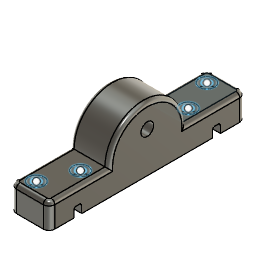
ersatzteilTischtennisplatte (Autodesk Fusion 360 design; units mm, degrees)
part number: 2025-12-14-13-54-51-674
Autodesk Fusion 360 part; units mm, degrees
sketch "Skizze1" plane through (0, 0, 0) normal (1, 0, 0) x (0, 1, 0)
  line L0 (0, 0) -> (51, 0)
  line L1 (0, 0) -> (-51, 0)
  line L2 (-51, 0) -> (-51, 13)
  line L3 (51, 0) -> (51, 13)
  line L4 (51, 13) -> (20, 13)
  line L5 (-51, 13) -> (-20, 13)
  arc A0 (20, 13) -> (-20, 13) centre (0, 13) ccw
  line L6 (-51, 0) -> (-38, 0)
  line L7 (51, 0) -> (38, 0)
  dimension "d6" = 13
  dimension "d10" = 51
  dimension "d11" = 40
  dimension "d12" = 13
  dimension "d13" = 13
  constraint coincident L0.start L1.start
  constraint horizontal L0
  constraint parallel L0 L1
  constraint perpendicular L1 L2
  constraint perpendicular L0 L3
  constraint perpendicular L3 L4
  constraint perpendicular L2 L5
  constraint perpendicular L2 L6
  constraint perpendicular L3 L7
  measures "d6" distance of L1.end L2.end
  measures "d10" distance of L0.start L0.end
  measures "d11" diameter of A0
  measures "d12" distance of L1.end L6.end
  measures "d13" distance of L0.end L7.end
extrude "Extrusion1" add sketch "Skizze1" along normal blind 20
fillet "Abrundung1" radius 2 8 edges at (10, -51, 13) (20, -35.5, 13) (0, -35.5, 13) (20, 0, 33) (0, 0, 33) (0, 35.5, 13) (20, 35.5, 13) (10, 51, 13)
fillet "Abrundung2" radius 3 8 edges at (0, 51, 5.5) (0.5858, 50.4142, 12.4142) (20, 51, 5.5) (19.4142, 50.4142, 12.4142) (19.4142, -50.4142, 12.4142) (20, -51, 5.5) (0, -51, 5.5) (0.5858, -50.4142, 12.4142)
sketch "Skizze2" plane through (20, 0, 0) normal (1, 0, 0) x (0, 1, 0)
  line L0 (-48, 11) -> (-48, 0)
  line L1 (-48, 0) -> (48, 0)
  line L2 (48, 0) -> (48, 11)
  line L3 (48, 11) -> (17.8885, 11)
  arc A0 (17.8885, 11) -> (-17.8885, 11) centre (0, 13) ccw
  line L4 (-17.8885, 11) -> (-48, 11)
  circle A1 centre (0, 21) radius 3.3
  dimension "d22" = 21
  dimension "d23" = 6.6
  measures "d22" distance of origin A1.centre
  measures "d23" diameter of A1
extrude "Extrusion2" cut sketch "Skizze2" against normal blind 100 contours A1
sketch "Skizze3" plane through (0, 0, 0) normal (-1, 0, 0) x (0, -1, 0)
  circle A0 centre (0, 21) radius 3.3
  line L0 (48, 0) -> (48, 11)
  line L1 (48, 11) -> (17.8885, 11)
  arc A1 (17.8885, 11) -> (-17.8885, 11) centre (0, 13) ccw
  line L2 (-17.8885, 11) -> (-48, 11)
  line L3 (-48, 11) -> (-48, 0)
  line L4 (-48, 0) -> (48, 0)
  line L5 (-6, 17.5359) -> (0, 14.0718)
  line L6 (0, 14.0718) -> (6, 17.5359)
  line L7 (6, 17.5359) -> (6, 24.4641)
  line L8 (6, 24.4641) -> (0, 27.9282)
  line L9 (0, 27.9282) -> (-6, 24.4641)
  line L10 (-6, 24.4641) -> (-6, 17.5359)
  point P0 (0, 21)
  dimension "d26" = 6
  constraint coincident P0 A0.centre
  measures "d26" distance of P0 L10
extrude "Extrusion3" cut sketch "Skizze3" against normal blind 6 contours L5 L6 L7 L8 L9 L10
sketch "Skizze4" plane through (0, 0, 0) normal (-1, 0, 0) x (0, -1, 0)
  line L0 (0, 14.0718) -> (-6, 17.5359)
  line L1 (-6, 17.5359) -> (-6, 24.4641)
  line L2 (-6, 24.4641) -> (0, 27.9282)
  line L3 (0, 27.9282) -> (6, 24.4641)
  line L4 (6, 24.4641) -> (6, 17.5359)
  line L5 (6, 17.5359) -> (0, 14.0718)
  line L6 (48, 0) -> (48, 11)
  line L7 (48, 11) -> (17.8885, 11)
  arc A0 (17.8885, 11) -> (-17.8885, 11) centre (0, 13) ccw
  line L8 (-17.8885, 11) -> (-48, 11)
  line L9 (-48, 11) -> (-48, 0)
  line L10 (-48, 0) -> (48, 0)
  line L11 (51, 0) -> (38, 0)
  line L12 (-51, 0) -> (-38, 0)
  line L13 (-38, 0) -> (-38, 4.8)
  line L14 (-38, 4.8) -> (-34, 4.8)
  line L15 (-34, 4.8) -> (-34, 0)
  dimension "d29" = 13
  dimension "d30" = 13
  dimension "d31" = 4.8
  dimension "d32" = 4
  constraint perpendicular L6 L11
  constraint perpendicular L9 L12
  constraint perpendicular L10 L13
  constraint perpendicular L13 L14
  constraint coincident L10 L15.end
  constraint perpendicular L10 L15
  measures "d29" distance of L11.start L11.end
  measures "d30" distance of L12.start L12.end
  measures "d31" distance of L12.end L13.end
  measures "d32" distance of L13.end L14.end
extrude "Extrusion4" cut sketch "Skizze4" against normal blind 100 contours L10 L13 L14 L15
fillet "Abrundung3" radius 1 2 edges at (10, 34, 4.8) (10, 38, 4.8)
sketch "Skizze5" plane through (0, 0, 0) normal (-1, 0, 0) x (0, -1, 0)
  line L0 (-34, 3.8) -> (-34, 0)
  line L1 (-34, 0) -> (48, 0)
  line L2 (48, 0) -> (48, 11)
  line L3 (48, 11) -> (17.8885, 11)
  arc A0 (17.8885, 11) -> (-17.8885, 11) centre (0, 13) ccw
  line L4 (-17.8885, 11) -> (-48, 11)
  line L5 (-48, 11) -> (-48, 0)
  line L6 (-48, 0) -> (-38, 0)
  line L7 (-38, 0) -> (-38, 3.8)
  arc A1 (-37, 4.8) -> (-38, 3.8) centre (-37, 3.8) ccw
  line L8 (-37, 4.8) -> (-35, 4.8)
  arc A2 (-34, 3.8) -> (-35, 4.8) centre (-35, 3.8) ccw
  line L9 (0, 14.0718) -> (-6, 17.5359)
  line L10 (-6, 17.5359) -> (-6, 24.4641)
  line L11 (-6, 24.4641) -> (0, 27.9282)
  line L12 (0, 27.9282) -> (6, 24.4641)
  line L13 (6, 24.4641) -> (6, 17.5359)
  line L14 (6, 17.5359) -> (0, 14.0718)
  line L15 (51, 0) -> (38, 0)
  line L16 (38, 0) -> (38, 4.8)
  line L17 (38, 4.8) -> (34, 4.8)
  line L18 (34, 4.8) -> (34, 0)
  dimension "d37" = 13
  dimension "d38" = 4.8
  dimension "d39" = 4
  constraint perpendicular L2 L15
  constraint perpendicular L1 L16
  constraint perpendicular L16 L17
  constraint coincident L1 L18.end
  constraint perpendicular L1 L18
  measures "d37" distance of L15.start L15.end
  measures "d38" distance of L15.end L16.end
  measures "d39" distance of L16.end L17.end
extrude "Extrusion5" cut sketch "Skizze5" against normal blind 100 contours L1 L16 L17 L18
fillet "Abrundung4" radius 1 2 edges at (10, -34, 4.8) (10, -38, 4.8)
sketch "Skizze6" plane through (0, 0, 13) normal (0, 0, 1) x (-1, 0, 0)
  arc A0 (-18, -48) -> (-17, -49) centre (-17, -48) ccw
  line L0 (-17, -49) -> (-3, -49)
  arc A1 (-3, -49) -> (-2, -48) centre (-3, -48) ccw
  line L1 (-2, -48) -> (-2, -20)
  line L2 (-2, -20) -> (-18, -20)
  line L3 (-18, -20) -> (-18, -48)
  circle A2 centre (-6.7, 44.3) radius 2.15
  circle A3 centre (-13.3, 28) radius 2.15
  circle A4 centre (-13.3, -28) radius 2.15
  circle A5 centre (-6.7, -44.3) radius 2.15
  circle A6 centre (-13.3, 28) radius 4
  circle A7 centre (-6.7, 44.3) radius 4
  circle A8 centre (-13.3, -28) radius 4
  circle A9 centre (-6.7, -44.3) radius 4
  dimension "d55" = 4.3
  dimension "d58" = 4.3
  dimension "d61" = 8
  dimension "d62" = 8
  dimension "d63" = 8
  dimension "d64" = 8
  dimension "d67" = 4.3
  dimension "d68" = 4.3
  constraint concentric A3 A6
  constraint concentric A2 A7
  constraint concentric A4 A8
  constraint concentric A5 A9
  measures "d55" diameter of A2
  measures "d58" diameter of A3
  measures "d61" diameter of A6
  measures "d62" diameter of A7
  measures "d63" diameter of A8
  measures "d64" diameter of A9
  measures "d67" diameter of A5
  measures "d68" diameter of A4
extrude "Extrusion6" cut sketch "Skizze6" against normal blind 100 contours A2 | A3 | A4 | A5
extrude "Extrusion7" cut sketch "Skizze6" against normal blind 4 contours A6 | A7 | A8 | A9
